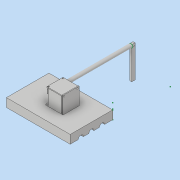
# Autodesk Inventor part: Vertical
Saved by Autodesk Inventor 2019 (Build 230136000, 136)
## iProperties
Created: 2020-02-15
Part Number: Vertical
Material: Generic
Document SubType Name: Modeling
Designer: Sudhanshu
Density: 1 g/cm^3
Appearance: Default
Author: Sudhanshu
Autodesk Inventor part; units mm, degrees
ref_plane "YZ Plane" through (0, 0, 0) normal (1, 0, 0) x (0, 1, 0)
ref_plane "XZ Plane" through (0, 0, 0) normal (0, 1, 0) x (-1, 0, 0)
ref_plane "XY Plane" through (0, 0, 0) normal (0, 0, 1) x (1, 0, 0)
sketch "Sketch1" plane through (0, 0, 0) normal (0, 1, 0) x (-1, 0, 0)
  line L0 (0, 0) -> (150, 0)
  line L1 (150, 0) -> (150, 100)
  line L2 (150, 100) -> (0, 100)
  line L3 (0, 100) -> (0, 0)
  dimension "d0" = 150
  dimension "d1" = 100
  constraints: 8 end point, 2 parallel, 1 horizontal, 1 perpendicular
  measures "d0" distance of L2.end L1.end
  measures "d1" distance of L1.end L0.end
extrude "Extrusion1" add sketch "Sketch1" along normal blind 20
sketch "Sketch2" plane through (0, 20, 0) normal (0, 1, 0) x (1, 0, 0)
  point P0 (0, 0)
sketch "Sketch3" plane through (0, 20, 0) normal (0, 1, 0) x (1, 0, 0)
  point P0 (0, 0)
sketch "Sketch4" plane through (0, 20, 0) normal (0, 1, 0) x (1, 0, 0)
  line L0 (-88.5149, -68.8546) -> (-50.8129, -68.8546)
  line L1 (-50.8129, -68.8546) -> (-50.8129, -31.4381)
  line L2 (-50.8129, -31.4381) -> (-88.5149, -31.4381)
  line L3 (-88.5149, -31.4381) -> (-88.5149, -68.8546)
  point P0 (0, 0)
  constraints: 8 end point, 2 parallel, 1 horizontal, 1 perpendicular
extrude "Extrusion2" add sketch "Sketch4" along normal blind 2
sketch "Sketch8" plane through (0, 22, 0) normal (0, 1, 0) x (1, 0, 0)
  point P0 (0, 0)
sketch "Sketch9" plane through (0, 22, 0) normal (0, 1, 0) x (1, 0, 0)
  line L0 (-50.8129, -68.8546) -> (-88.5149, -68.8546) projected
  line L1 (-88.5149, -31.4381) -> (-50.8129, -31.4381) projected
  line L2 (-82.8248, -68.8546) -> (-52.6097, -68.8546)
  line L3 (-52.6097, -68.8546) -> (-52.6097, -31.4381)
  line L4 (-52.6097, -31.4381) -> (-82.8248, -31.4381)
  line L5 (-82.8248, -31.4381) -> (-82.8248, -68.8546)
  point P0 (0, 0)
  constraints: 8 end point, 2 parallel, 2 point on line, 1 horizontal, 1 perpendicular
extrude "Extrusion5" add sketch "Sketch9" along normal blind 35
sketch "Sketch10" plane through (-82.8248, 22, 31.4381) normal (-1, 0, 0) x (0, 0, 1)
  line L0 (13.2287, 19.9432) -> (24.5588, 19.9432)
  line L1 (24.5588, 19.9432) -> (24.5588, 10.3562)
  line L2 (24.5588, 10.3562) -> (13.2287, 10.3562)
  line L3 (13.2287, 10.3562) -> (13.2287, 19.9432)
  point P0 (-31.4381, -22)
  constraints: 8 end point, 2 parallel, 1 horizontal, 1 perpendicular
extrude "Extrusion6" add sketch "Sketch10" along normal blind 15
sketch "Sketch12" plane through (-82.8248, 32.3562, 44.6668) normal (0, 0, -1) x (-1, 0, 0)
  circle A0 centre (10.1482, 4.7576) radius 4.2682
  point P0 (-82.8248, -32.3562)
  constraints: 1 centre point
extrude "Extrusion7" add sketch "Sketch12" along normal blind 180
sketch "Sketch13" plane through (-97.8248, 22, 31.4381) normal (-1, 0, 0) x (0, 0, 1)
  point P0 (-31.4381, -22)
sketch "Sketch14" plane through (0, 0, 0) normal (0, 0, 1) x (1, 0, 0)
  point P0 (0, 0)
sketch "Sketch15" plane through (0, 0, 0) normal (0, 1, 0) x (-1, 0, 0)
  point P0 (0, 0)
sketch "Sketch16" plane through (0, 0, 0) normal (0, 1, 0) x (-1, 0, 0)
  point P0 (0, 0)
sketch "Sketch17" plane through (-92.973, 37.1137, -135.3332) normal (0, 0, -1) x (-1, 0, 0)
  circle A0 centre (0, 0) radius 4.2682 projected
  point P0 (-92.973, -37.1137)
sketch "Sketch18" plane through (-92.973, 37.1137, -135.3332) normal (0, 0, -1) x (-1, 0, 0)
  point P0 (-92.973, -37.1137)
sketch "Sketch19" plane through (-92.973, 37.1137, -135.3332) normal (0, 0, -1) x (-1, 0, 0)
  point P0 (-92.973, -37.1137)
sketch "Sketch20" plane through (-92.973, 37.1137, -135.3332) normal (0, 0, -1) x (-1, 0, 0)
  line L0 (-2.448, 2.726) -> (2.3625, 2.726)
  line L1 (2.3625, 2.726) -> (2.3625, -2.6968)
  line L2 (2.3625, -2.6968) -> (-2.448, -2.6968)
  line L3 (-2.448, -2.6968) -> (-2.448, 2.726)
  point P0 (-92.973, -37.1137)
  constraints: 8 end point, 2 parallel, 1 horizontal, 1 perpendicular
extrude "Extrusion8" add sketch "Sketch20" along normal blind 8
sketch "Sketch21" plane through (-95.3355, 34.417, -135.3332) normal (0, -1, 0) x (1, 0, 0)
  point P0 (95.3355, 135.3332)
sketch "Sketch22" plane through (-95.3355, 34.417, -135.3332) normal (0, -1, 0) x (1, 0, 0)
  point P0 (95.3355, 135.3332)
sketch "Sketch23" plane through (-95.3355, 34.417, -135.3332) normal (0, -1, 0) x (1, 0, 0)
  line L0 (0, -8) -> (4.8105, -8) projected
  line L1 (-1.9057, 0) -> (6.6307, 0) projected
  line L2 (0, -8) -> (4.9417, -8)
  line L3 (4.9417, -8) -> (4.9417, 0)
  line L4 (4.9417, 0) -> (0, 0)
  line L5 (0, 0) -> (0, -8)
  point P0 (95.3355, 135.3332)
  constraints: 8 end point, 2 parallel, 1 horizontal, 1 perpendicular, 1 point on line
extrude "Extrusion9" add sketch "Sketch23" along normal blind 70
sketch "Sketch27" plane through (0, 0, 100) normal (1, 0, 0) x (0, 0, -1)
  line L0 (0, 0) -> (100, 0)
  line L1 (100, 0) -> (50, 0)
  line L2 (100, 0) -> (0, 0) projected
  line L3 (75, 0) -> (50, 0)
  line L4 (0, 0) -> (50, 0)
  circle A0 centre (25, 0) radius 6
  circle A1 centre (50, 0) radius 6
  circle A2 centre (75, 0) radius 6
  dimension "d24" = 12
  dimension "d25" = 12
  dimension "d26" = 12
  constraints: 8 end point, 3 centre point, 3 midpoint, 2 coincident, 2 collinear, 1 horizontal
  measures "d24" diameter of A0
  measures "d25" diameter of A1
  measures "d26" diameter of A2
extrude "Extrusion10" cut sketch "Sketch27" along normal through all both and the other way through all
sketch "Sketch30" plane through (0, 57, 0) normal (0, 1, 0) x (1, 0, 0)
  line L0 (-150, -31) -> (0, -31) projected
  line L1 (-85.8103, -31) -> (-48.4742, -31)
  line L2 (-48.4742, -31) -> (-48.4742, -68.8679)
  line L3 (-48.4742, -68.8679) -> (-85.8103, -68.8679)
  line L4 (-85.8103, -68.8679) -> (-85.8103, -31)
  point P0 (0, 0)
  constraints: 8 end point, 2 parallel, 1 horizontal, 1 perpendicular, 1 point on line
extrude "Extrusion11" add sketch "Sketch30" along normal blind 2
sketch "Sketch31" plane through (0, 20, 0) normal (0, 1, 0) x (1, 0, 0)
  line L0 (0, -69) -> (-150, -69) projected
  line L1 (-150, -31) -> (0, -31) projected
  line L2 (-49.8943, -69) -> (-47.9179, -69)
  line L3 (-47.9179, -69) -> (-47.9179, -31)
  line L4 (-47.9179, -31) -> (-49.8943, -31)
  line L5 (-49.8943, -31) -> (-49.8943, -69)
  point P0 (0, 0)
  constraints: 8 end point, 2 parallel, 2 point on line, 1 horizontal, 1 perpendicular
extrude "Extrusion12" add sketch "Sketch31" along normal blind 40
sketch "Sketch32" plane through (0, 59, 0) normal (0, 1, 0) x (1, 0, 0)
  circle A0 centre (-83.7761, -33.1539) radius 1.2799
  circle A1 centre (-83.7761, -66.902) radius 1.3017
  point P0 (0, 0)
  constraints: 2 centre point
extrude "Extrusion13" cut sketch "Sketch32" against normal blind 40
sketch "Sketch33" plane through (-47.9179, 20, 69) normal (1, 0, 0) x (0, 0, -1)
  line L0 (0.1321, 37) -> (38, 37) projected
  circle A0 centre (34.1824, 37) radius 1.5602
  circle A1 centre (2.8109, 37) radius 1.6636
  point P0 (69, -20)
  constraints: 2 centre point, 1 point on line
extrude "Extrusion14" cut sketch "Sketch33" against normal blind 40
body "Solid1"
